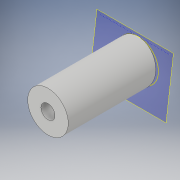
# Autodesk Inventor part: HoleFill1
Saved by Autodesk Inventor 2019 (Build 230136000, 136)
## iProperties
Created: 2019-04-21
Part Number: HoleFill1
Material: Generic
Document SubType Name: Modeling
Designer: lgnds
Density: 1 g/cm^3
Appearance: Default
Author: lgnds
Autodesk Inventor part; units mm, degrees
ref_plane "YZ Plane" through (0, 0, 0) normal (1, 0, 0) x (0, 1, 0)
ref_plane "XZ Plane" through (0, 0, 0) normal (0, 1, 0) x (-1, 0, 0)
ref_plane "XY Plane" through (0, 0, 0) normal (0, 0, 1) x (1, 0, 0)
sketch "Sketch1" plane through (0, 0, 0) normal (0, 0, 1) x (1, 0, 0)
  circle A0 centre (0, 0) radius 7.2
  dimension "d0" = 14.4
  constraints: 1 centre point, 1 coincident
  measures "d0" diameter of A0
extrude "Extrusion1" add sketch "Sketch1" along normal blind 32
sketch "Sketch2" plane through (0, 0, 32) normal (0, 0, 1) x (1, 0, 0)
  circle A0 centre (0, 0) radius 2.5
  dimension "d3" = 5
  constraints: 1 centre point, 1 coincident
  measures "d3" diameter of A0
extrude "Extrusion2" cut sketch "Sketch2" against normal blind 10
sketch "Sketch3" plane through (0, 0, 0) normal (0, 0, 1) x (1, 0, 0)
  circle A0 centre (0, 0) radius 7.2 projected
  line L0 (11.2434, 7.2) -> (-13.4853, 7.2) construction
  constraints: 2 end point, 1 horizontal, 1 tangent
ref_plane "Work Plane1" through (11.2434, 7.2, 0) normal (0, -0.1297, -0.9916) x (-1, 0, 0)
sketch "Sketch4" plane through (11.2434, 7.2, 0) normal (0, -0.1297, -0.9916) x (-1, 0, 0)
  line L0 (30.8181, -24.4459) -> (-8.3313, -24.4459)
  line L1 (-8.3313, -24.4459) -> (-8.3313, 10.1675)
  line L2 (-8.3313, 10.1675) -> (30.8181, 10.1675)
  line L3 (30.8181, 10.1675) -> (30.8181, -24.4459)
  line L4 (30.8181, -24.4459) -> (-8.3313, 10.1675) construction
  line L5 (-8.3313, -24.4459) -> (30.8181, 10.1675) construction
  point P0 (11.2434, -7.1392)
  constraints: 12 end point, 2 midpoint, 2 parallel, 1 horizontal, 1 perpendicular
extrude "Extrusion3" cut sketch "Sketch4" along normal blind 10
body "Solid1"
